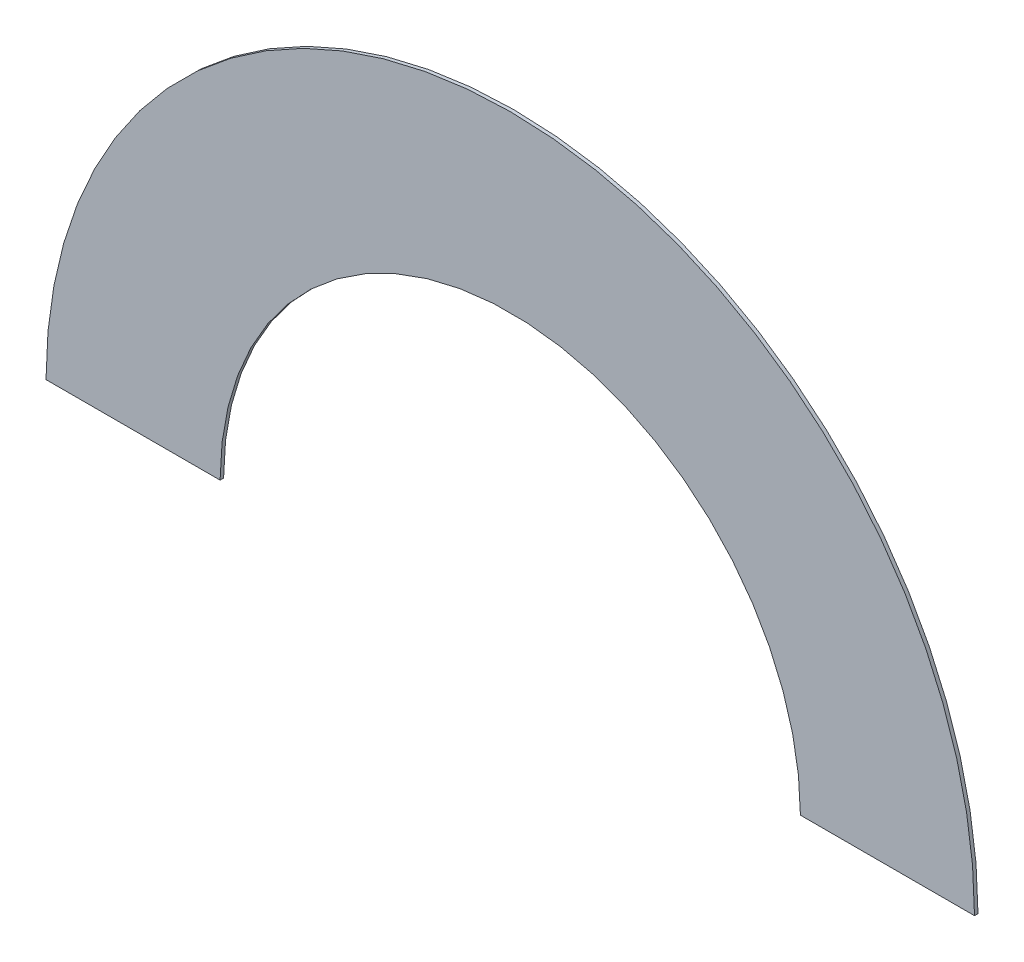
# Autodesk Inventor part: RingWhite
Saved by Autodesk Inventor 2025.2 (Build 292293000, 293)
## iProperties
Created: 2024-11-19
Part Number: RingWhite
Material: Generic
Document SubType Name: Modeling
Designer: jaros
Density: 1 g/cm^3
Appearance: Default
Author: jaros
Autodesk Inventor part; units mm, degrees
ref_plane "YZ Plane" through (0, 0, 0) normal (1, 0, 0) x (0, 1, 0)
ref_plane "XZ Plane" through (0, 0, 0) normal (0, 1, 0) x (-1, 0, 0)
ref_plane "XY Plane" through (0, 0, 0) normal (0, 0, 1) x (1, 0, 0)
ref_plane "Work Plane1" through (0, 0, -3) normal (0, 0, -1) x (-1, 0, 0)
sketch "Sketch1" plane through (0, 0, -3) normal (0, 0, -1) x (-1, 0, 0)
  circle A0 centre (0, 0) radius 250 construction
  arc A1 (250, 0) -> (-250, 0) centre (0, 0) ccw
  arc A2 (400, 0) -> (-400, 0) centre (0, 0) ccw
  line L0 (250, 0) -> (400, 0)
  line L1 (-250, 0) -> (-400, 0)
  dimension "d0" = 150
  constraints: 7 point on circle, 4 end point, 2 centre point, 2 horizontal, 1 concentric
  measures "d0" distance of L0.start L0.end
extrude "Extrusion1" add sketch "Sketch1" against normal blind 3
body "Solid1"
